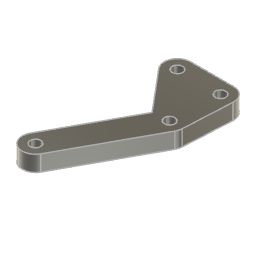
_ConnectorArm.6e87e7e7-3f8f-4d0b-aee9-b19efa5eba7e (Autodesk Fusion 360 design; units mm, degrees)
Autodesk Fusion 360 part; units mm, degrees
other "Derived from MasterParameters_Gripper v69"
sketch "Sketch1" plane through (0, 0, 0) normal (0, 0, 1) x (1, 0, 0)
  circle A0 centre (0, 0) radius 3.35
  circle A1 centre (-12, -22) radius 3.35
  circle A2 centre (-12, -22) radius 1.35
  circle A3 centre (0, 0) radius 1.35
  line L0 (2.941, -1.6042) -> (-9.059, -23.6042)
  line L1 (-2.941, 1.6042) -> (-14.941, -20.3958)
  circle A4 centre (0.65, 12.2554) radius 3.35
  circle A5 centre (-10.2734, 12.2554) radius 3.35
  line L2 (3.3453, -0.1774) -> (3.9953, 12.078)
  line L3 (0.65, 15.6054) -> (-10.2734, 15.6054)
  line L4 (-10.2734, 8.9054) -> (0.65, 8.9054)
  line L5 (-7.7061, 14.4075) -> (2.5673, 2.1521)
  line L6 (-12.8407, 10.1033) -> (-2.5673, -2.1521)
  line L7 (-2.6953, 12.4328) -> (-3.4568, -1.9249)
  circle A6 centre (0.65, 12.2554) radius 1.35
  circle A7 centre (-10.2734, 12.2554) radius 1.35
  point P0 (4, 12.2554)
  constraint coincident A0.centre A3.centre
  constraint concentric A1 A2
  constraint equal A2 A3
  constraint equal A0 A1
  constraint coincident A0 L0.start
  constraint coincident A1 L0.end
  constraint tangent A1 L0
  constraint coincident A0 L1.start
  constraint coincident A1 L1.end
  constraint tangent A1 L1
  constraint tangent A0 L1
  constraint tangent A0 L0
  constraint coincident A4 P0
  constraint horizontal A4.centre P0
  constraint equal A0 A4
  constraint equal A0 A5
  constraint horizontal A4.centre A5.centre
  constraint coincident A0 L2.start
  constraint coincident A4 L2.end
  constraint tangent A4 L2
  constraint coincident A4 L3.start
  constraint coincident A5 L3.end
  constraint tangent A4 L3
  constraint tangent A5 L3
  constraint coincident A5 L4.start
  constraint coincident A4 L4.end
  constraint tangent A4 L4
  constraint tangent A5 L4
  constraint coincident A5 L5.start
  constraint coincident A0 L5.end
  constraint coincident A5 L6.start
  constraint coincident A0 L6.end
  constraint tangent A0 L6
  constraint tangent A5 L6
  constraint tangent A5 L5
  constraint tangent A0 L5
  constraint coincident A4 L7.start
  constraint tangent A0 L7
  constraint tangent A4 L7
  constraint concentric A4 A6
  constraint concentric A5 A7
  constraint equal A3 A6
  constraint equal A3 A7
  constraint tangent A0 L2
  measures "d1" distance of A0.centre A1.centre
  measures "d30" diameter of A3
  measures "d31" distance of A1 A2
  measures "d32" distance of A1.centre A0.centre
  measures "d45" distance of A0.centre P0
extrude "Extrude1" add sketch "Sketch1" along normal blind 4
equation "d1 = plate_distance_back_front_y_Ref"
equation "m2_nut_diameter_Ref = 4.2 mm"
equation "m2_nut_height_Ref = 3 mm"
equation "arm_screw_wall_thickness_Ref = 1 mm"
equation "m2_screw_diameter_Ref = 2.2 mm" comment "diameter with tolerance"
equation "m25_screw_diameter_Ref = 2.7 mm"
equation "m25_wall_thickness_Ref = 2 mm"
equation "m2_tapping_tolerance_Ref = 0.2 mm"
equation "Servo_cut_gap_Ref = 0.5 mm"
equation "m25_screw_head_height_Ref = 2.5 mm"
equation "m25_screw_head_width_Ref = 4.6 mm"
equation "m25_arm_screw_plus_tolerance_Ref = 2.9 mm" comment "Additional parameter to experiment with parameter to hopefully enable free movement of arm"
equation "m2_tapping_head_width_Ref = 4.4 mm"
equation "back_arms_thickness_Ref = 8.5 mm"
equation "m2_screw_head_diameter_Ref = 4 mm"
equation "m2_screw_head_height_Ref = 2 mm"
equation "arm_height_Ref = 4 mm"
equation "arm_ground_clearance_Ref = 1 mm"
equation "m3_screw_diameter_Ref = 3.2 mm"
equation "m3_wall_thickness_gripper_mount_Ref = 2 mm"
equation "arm_length_Ref = 27.5 mm"
equation "gear_arm_gap_Ref = 0.05 mm"
equation "distance_lower_upper_plate_Ref = 10 mm"
equation "gear_screw_dist_Ref = 1.5 mm"
equation "gear_z_height_placement_on_arm_Ref = 5 mm"
equation "plate_distance_back_axes_Ref = 30 mm" comment "Distance between back-axes, namely servo and the arm axis of the arm in the back"
equation "distance_arms_front_Ref = 12 mm" comment "Distance from the back to the front axis"
equation "d30 = m25_screw_diameter_Ref"
equation "d31 = m25_wall_thickness_Ref"
equation "d32 = distance_arms_front_Ref"
equation "d33 = arm_height_Ref"
equation "gear_arm_connector_height_Ref = 4 mm"
equation "m25_ruthex_outer_Ref = 7.2 mm"
equation "m25_ruthex_inner_Ref = 4 mm"
equation "m25_ruthex_height_Ref = 5.7 mm"
equation "plate_single_height_Ref = 3 mm" comment "height of a single plate piece"
equation "plate_distance_back_front_y_Ref = 22 mm"
equation "stand_width_Ref = 5 mm" comment "width of the stand that the gripper can be mounted onto"
equation "gripper_tpu_thickness_Ref = 6 mm"
equation "arm_top_tolerance_Ref = 0.2 mm"
equation "gear_square_length_Ref = 5.9 mm"
equation "m25_nyloc_width_Ref = 5.2 mm"
equation "m25_nyloc_height_Ref = 3.8 mm"
